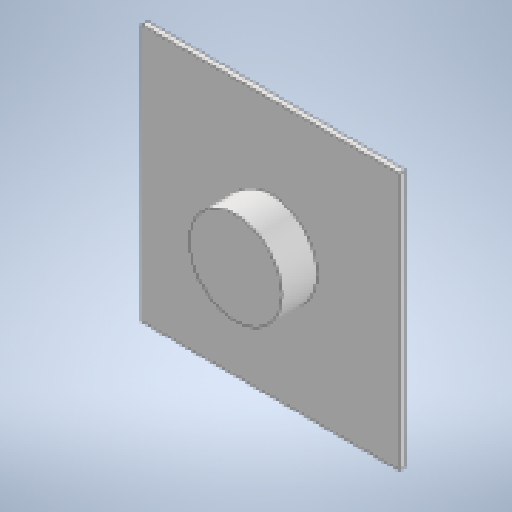
# Autodesk Inventor part: Acrilico_Top
Saved by Autodesk Inventor 2024 (Build 280153000, 153)
## iProperties
Created: 2023-06-28
Part Number: Acrilico_Top
Material: Genérico
Document SubType Name: Modeling
Designer: Personal
Mass: 247.6 g
Surface Area: 853.097 cm^2
Volume: 269.294 cm^3
Density: 0.919441 g/cm^3
Appearance: Valor por defecto
Author: Personal
Autodesk Inventor part; units mm, degrees
ref_plane "YZ Plane" through (0, 0, 0) normal (1, 0, 0) x (0, 1, 0)
ref_plane "XZ Plane" through (0, 0, 0) normal (0, 1, 0) x (-1, 0, 0)
ref_plane "XY Plane" through (0, 0, 0) normal (0, 0, 1) x (1, 0, 0)
sketch "Boceto1" plane through (0, 0, 0) normal (0, 0, 1) x (1, 0, 0)
  line L0 (186.1, 8.9) -> (186.1, -186.1) projected
  line L1 (-8.9, 8.9) -> (-8.9, -186.1) projected
  line L2 (186.1, -186.1) -> (-8.9, -186.1)
  line L3 (-8.9, 8.9) -> (186.1, 8.9)
  point P0 (0, 0)
  constraints: 4 end point, 1 horizontal, 1 parallel
extrude "Extrusión1" add sketch "Boceto1" along normal blind 4.4
sketch "Boceto2" plane through (0, 0, 4.4) normal (0, 0, 1) x (1, 0, 0)
  line L0 (186.1, -186.1) -> (186.1, 8.9) projected
  line L1 (-8.9, -186.1) -> (186.1, -186.1) projected
  line L2 (-8.9, 8.9) -> (-8.9, -186.1) projected
  line L3 (186.1, 8.9) -> (-8.9, 8.9) projected
  circle A0 centre (88.6021, -88.6021) radius 35
  point P0 (0, 0)
  dimension "d2" = 70
  dimension "d3" = 97.4979
  dimension "d4" = 97.4979
  constraints: 1 centre point
  measures "d2" diameter of A0
  measures "d3" distance from line of L0 A0.centre
  measures "d4" distance from line of L1 A0.centre
extrude "Extrusión2" add sketch "Boceto2" along normal blind 26.5 contours A0
